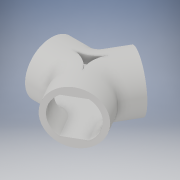
# Autodesk Inventor part: 3 way corridor
Saved by Autodesk Inventor 2017 (Build 210142000, 142)
## iProperties
Created: 2018-03-04
Part Number: 3 way corridor
Material: Generic
Document SubType Name: Modeling
Designer: Braxton
Density: 1 g/cm^3
Appearance: Default
Author: Braxton
Autodesk Inventor part; units mm, degrees
ref_plane "YZ Plane" through (0, 0, 0) normal (1, 0, 0) x (0, 1, 0)
ref_plane "XZ Plane" through (0, 0, 0) normal (0, 1, 0) x (-1, 0, 0)
ref_plane "XY Plane" through (0, 0, 0) normal (0, 0, 1) x (1, 0, 0)
sketch "Sketch1" plane through (0, 0, 0) normal (1, 0, 0) x (0, 1, 0)
  line L0 (84.6667, 50.8) -> (84.6667, -50.8)
  line L1 (-84.6667, 50.8) -> (-84.6667, -50.8)
  circle A0 centre (0, 0) radius 124.1375
  arc A1 (84.6667, 50.8) -> (-84.6667, 50.8) centre (0, 0) ccw
  arc A2 (-84.6667, -50.8) -> (84.6667, -50.8) centre (0, 0) ccw
  dimension "d10" = 169.3333
  dimension "d11" = 101.6
  dimension "d14" = 248.2749
  constraints: 4 end point, 4 point on circle, 3 centre point, 2 coincident, 1 parallel
  measures "d10" distance between parallel lines of L1 L0
  measures "d11" distance of L0.start L0.end
  measures "d14" diameter of A0
extrude "corridor" add sketch "Sketch1" along normal blind 101.6
sketch "found rotaion axis" plane through (0, 0, 0) normal (0, 1, 0) x (-1, 0, 0)
  line L0 (-101.6, 124.1375) -> (-101.6, -124.1375) projected
  line L1 (-101.6, -124.1375) -> (-101.6, 124.1375)
  line L2 (-101.6, 0) -> (-173.2708, 0)
  point P0 (0, 0)
  dimension "d15" = 71.6708
  constraints: 4 end point, 1 horizontal, 1 midpoint, 1 vertical
  measures "d15" distance of L2.start L2.end
pattern_circular "other corridors" count 3 over 360 about axis through (173.2708, 0, 0) along (0, 1, 0) of "corridor"
sketch "Sketch4" plane through (0, 0, 0) normal (0, 1, 0) x (-1, 0, 0)
  line L0 (0, -98.7375) -> (-101.6, -98.7375) projected
  line L1 (-174.397, -199.4256) -> (-123.597, -111.4375) projected
  line L2 (-101.6, -98.7375) -> (0, -98.7375)
  line L3 (0, -124.1375) -> (0, 124.1375) projected
  line L4 (-123.597, -111.4375) -> (-174.397, -199.4256)
  line L5 (-367.4124, -87.9882) -> (-152.4, -212.1256) projected
  line L6 (-345.4153, -100.6882) -> (-294.6153, -12.7) projected
  line L7 (-345.4153, -100.6882) -> (-294.6153, -12.7)
  line L8 (-345.4153, 100.6882) -> (-294.6153, 12.7) projected
  line L9 (-294.6153, 12.7) -> (-345.4153, 100.6882)
  line L10 (-174.397, 199.4256) -> (-123.597, 111.4375) projected
  line L11 (-123.597, 111.4375) -> (-165.1121, 87.4687) projected
  line L12 (-174.397, 199.4256) -> (-123.597, 111.4375)
  line L13 (0, 98.7375) -> (-101.6, 98.7375) projected
  line L14 (-101.6, 98.7375) -> (0, 98.7375)
  line L15 (-101.6, -124.1375) -> (-316.6124, 0) projected
  arc A0 (-101.6, -98.7375) -> (-123.597, -111.4375) centre (-101.6, -124.1375) ccw
  arc A1 (-294.6153, -12.7) -> (-294.6153, 12.7) centre (-316.6124, 0) ccw
  line L16 (-316.6124, 0) -> (-101.6, 124.1375) projected
  arc A2 (-123.597, 111.4375) -> (-101.6, 98.7375) centre (-101.6, 124.1375) ccw
  point P0 (0, 0)
  constraints: 13 end point, 11 point on line, 8 point on circle, 3 centre point, 3 perpendicular, 1 coincident
sketch "Sketch5" plane through (101.6, 0, 0) normal (1, 0, 0) x (0, 0, -1)
  arc A0 (50.8, -84.6667) -> (50.8, 84.6667) centre (0, 0) ccw
  arc A1 (0, -124.1375) -> (0, 124.1375) centre (0, 0) ccw
  line L0 (50.8, 84.6667) -> (0, 84.6667)
  line L1 (50.8, -84.6667) -> (0, -84.6667)
  line L2 (0, 124.1375) -> (0, 84.6667)
  line L3 (0, -84.6667) -> (0, -124.1375)
  constraints: 8 end point, 4 point on circle, 2 centre point, 2 coincident, 2 point on line, 2 vertical
sweep "curve edjes" add profiles "Sketch5" path "Sketch4" path curves A0
pattern_circular "repeat curve edjes" count 3 over 360 about axis through (173.2708, 0, 0) along (0, 1, 0) of "curve edjes"
sketch "Sketch7" plane through (0, -84.6667, 50.8) normal (0, 1, 0) x (1, 0, 0)
  arc A0 (209.1062, -11.2687) -> (101.6, 50.8) centre (101.6, -73.3375) ccw projected
  arc A1 (209.1062, -11.2687) -> (101.6, 50.8) centre (101.6, -73.3375) ccw
  arc A2 (101.6, 50.8) -> (209.1062, 112.8687) centre (101.6, 174.9375) ccw projected
  line L0 (316.6124, 50.8) -> (209.1062, -11.2687) projected
  arc A3 (209.1062, 112.8687) -> (209.1062, -11.2687) centre (316.6124, 50.8) ccw
  arc A4 (209.1062, 112.8687) -> (209.1062, -11.2687) centre (316.6124, 50.8) ccw projected
  line L1 (209.1062, 112.8687) -> (316.6124, 50.8) projected
  arc A5 (101.6, 50.8) -> (209.1062, 112.8687) centre (101.6, 174.9375) ccw
  point P0 (173.2708, 50.8)
  constraints: 6 point on circle, 3 centre point, 3 concentric
extrude "Extrusion2" add sketch "Sketch7" against normal blind 39.4708 contours A0 A2 A3
body "Solid1"
